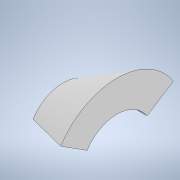
# Autodesk Inventor part: brake
Saved by Autodesk Inventor 2021.1 (Build 251245000, 245)
## iProperties
Created: 2020-08-18
Part Number: brake
Material: Generic
Document SubType Name: Modeling
Designer: robst
Density: 1 g/cm^3
Appearance: Default
Author: robst
Autodesk Inventor part; units mm, degrees
ref_plane "YZ Plane" through (0, 0, 0) normal (1, 0, 0) x (0, 1, 0)
ref_plane "XZ Plane" through (0, 0, 0) normal (0, 1, 0) x (-1, 0, 0)
ref_plane "XY Plane" through (0, 0, 0) normal (0, 0, 1) x (1, 0, 0)
sketch "Sketch1" plane through (0, 0, 0) normal (0, 0, 1) x (1, 0, 0)
  line L0 (0, 7.9375) -> (12.0984, 7.9375)
  line L1 (0, 7.9375) -> (12.0984, 14.9225)
  line L2 (12.0984, 14.9225) -> (12.0984, 7.9375)
  line L3 (0, 0) -> (25.4, 0) construction
  line L4 (0, 0) -> (0, 7.9375) construction
  dimension "d1" = 7.9375
  dimension "d3" = 30
  dimension "d7" = 6.985
  constraints: 10 end point, 2 horizontal, 2 vertical
  measures "d1" distance from line of L0 L3.start
  measures "d3" angle of L1 L0
  measures "d7" vertical distance of L1.end L0.start
revolve "Revolution1" add sketch "Sketch1" angle 115 mid plane about axis through (0, 0, 0) along (1, 0, 0)
body "Solid1"
